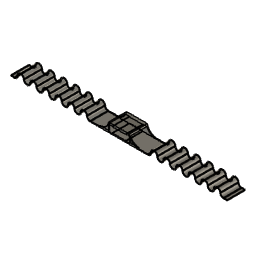
ACUTE_Prototype 3 v1 (Autodesk Fusion 360 design; units mm, degrees)
Autodesk Fusion 360 part; units mm, degrees
note: some values were not read from the file. Set by a fixed rule: which sketch regions a step uses.
sketch "Sketch1" plane through (0, 0, 0) normal (0, 0, 1) x (1, 0, 0)
  line L0 (0, 0) -> (240, 0)
  line L1 (240, 0) -> (240, 20)
  line L2 (240, 20) -> (0, 20)
  line L3 (0, 20) -> (0, 0)
  line L4 (120, 0) -> (120, 20) construction
  line L5 (130, 20) -> (110, 20)
  line L6 (110, 20) -> (110, 0)
  line L7 (110, 0) -> (130, 0)
  line L8 (130, 0) -> (130, 20)
  line L9 (130, 20) -> (110, 0) construction
  line L10 (110, 20) -> (130, 0) construction
  line L11 (127.5, 19) -> (112.5, 19)
  line L12 (112.5, 19) -> (112.5, 1)
  line L13 (112.5, 1) -> (127.5, 1)
  line L14 (127.5, 1) -> (127.5, 19)
  line L15 (127.5, 19) -> (112.5, 1) construction
  line L16 (112.5, 19) -> (127.5, 1) construction
  point P0 (120, 10)
  point P1 (120, 10)
  dimension "d1" = 240
  dimension "d2" = 20
  dimension "d3" = 20
  dimension "d4" = 15
  dimension "d5" = 18
  constraint horizontal L0
  constraint vertical L1
  constraint horizontal L2
  constraint vertical L3
  constraint coincident L0.start L3.end
  constraint midpoint L0 L4.start
  constraint midpoint L2 L4.end
  constraint horizontal L5
  constraint perpendicular L5 L6
  constraint parallel L5 L7
  constraint parallel L6 L8
  constraint coincident L9 P1
  constraint coincident L10 P1
  constraint midpoint L4 P1
  constraint horizontal L11
  constraint perpendicular L11 L12
  constraint parallel L11 L13
  constraint parallel L12 L14
  constraint coincident L15 P1
  constraint coincident L16 P1
  constraint coincident P1 P0
  measures "d1" distance of L0.start L0.end
  measures "d2" distance of L0.start L2.end
  measures "d3" distance of L6.end L7.end
  measures "d4" distance of L12.end L13.end
  measures "d5" distance of L11.end L12.end
extrude "Extrude1" add sketch "Sketch1" along normal blind 10 contours L0 L2 L3 L6 | L0 L2 L5 L6 L7 L8 | L0 L1 L2 L8 | L11 L12 L13 L14
sketch "Sketch2" plane through (0, 0, 0) normal (0, -1, 0) x (1, 0, 0)
  line L0 (0, 0) -> (240, 0)
  line L1 (240, 0) -> (240, 10)
  line L2 (240, 10) -> (0, 10)
  line L3 (0, 10) -> (0, 0)
  line L4 (0, 4) -> (100, 4) construction
  arc A0 (4, 1) -> (7, 4) centre (4, 4) ccw
  arc A1 (4, 0) -> (8, 4) centre (4, 4) ccw
  arc A2 (15, 4) -> (7, 4) centre (11, 4) ccw
  arc A3 (14, 4) -> (8, 4) centre (11, 4) ccw
  arc A4 (14, 4) -> (22, 4) centre (18, 4) ccw
  arc A5 (15, 4) -> (21, 4) centre (18, 4) ccw
  arc A6 (29, 4) -> (21, 4) centre (25, 4) ccw
  arc A7 (28, 4) -> (22, 4) centre (25, 4) ccw
  arc A8 (28, 4) -> (36, 4) centre (32, 4) ccw
  arc A9 (29, 4) -> (35, 4) centre (32, 4) ccw
  arc A10 (43, 4) -> (35, 4) centre (39, 4) ccw
  arc A11 (42, 4) -> (36, 4) centre (39, 4) ccw
  arc A12 (42, 4) -> (50, 4) centre (46, 4) ccw
  arc A13 (43, 4) -> (49, 4) centre (46, 4) ccw
  arc A14 (57, 4) -> (49, 4) centre (53, 4) ccw
  arc A15 (56, 4) -> (50, 4) centre (53, 4) ccw
  arc A16 (56, 4) -> (64, 4) centre (60, 4) ccw
  arc A17 (57, 4) -> (63, 4) centre (60, 4) ccw
  arc A18 (71, 4) -> (63, 4) centre (67, 4) ccw
  arc A19 (70, 4) -> (64, 4) centre (67, 4) ccw
  arc A20 (70, 4) -> (78, 4) centre (74, 4) ccw
  arc A21 (71, 4) -> (77, 4) centre (74, 4) ccw
  arc A22 (85, 4) -> (77, 4) centre (81, 4) ccw
  arc A23 (84, 4) -> (78, 4) centre (81, 4) ccw
  line L5 (0, 0) -> (0, 1) construction
  line L6 (0, 1) -> (98.101, 1) construction
  line L7 (98.101, 1) -> (88, 1)
  arc A24 (85, 4) -> (88, 1) centre (88, 4) ccw
  arc A25 (84, 4) -> (88, 0) centre (88, 4) ccw
  line L8 (4, 1) -> (0, 1)
  line L9 (4, 0) -> (0, 0)
  line L10 (98.101, 1) -> (98.101, 0)
  line L11 (120, 10) -> (120, 0) construction
  line L12 (131.5, 10) -> (108.5, 10)
  line L13 (108.5, 10) -> (108.5, 0)
  line L14 (108.5, 0) -> (131.5, 0)
  line L15 (131.5, 0) -> (131.5, 10)
  line L16 (131.5, 10) -> (108.5, 0) construction
  line L17 (108.5, 10) -> (131.5, 0) construction
  arc A26 (98.101, 1) -> (108.5, 10) centre (98.101, 11.5078) ccw
  point P0 (120, 5)
  dimension "d53" = 4
  dimension "d55" = 8
  dimension "d56" = 6
  dimension "d57" = 8
  dimension "d58" = 6
  dimension "d65" = 1
  dimension "d66" = 8
  dimension "d67" = 6
  dimension "d73" = 23
  constraint coincident L3 L4.start
  constraint concentric A0 A1
  constraint concentric A2 A3
  constraint tangent A0 A2
  constraint tangent A3 A4
  constraint tangent L3 A1
  constraint coincident L4 A0.end
  constraint coincident L4 A1.end
  constraint coincident L4 A3.start
  constraint coincident L4 A5.end
  constraint coincident L4 A2.start
  constraint coincident L4 A4.end
  constraint coincident L4 A7.start
  constraint coincident L4 A6.start
  constraint coincident L4 A9.end
  constraint coincident L4 A8.end
  constraint coincident L4 A11.start
  constraint coincident L4 A10.start
  constraint coincident L4 A13.end
  constraint coincident L4 A12.end
  constraint coincident L4 A15.start
  constraint coincident L4 A14.start
  constraint coincident L4 A17.end
  constraint coincident L4 A16.end
  constraint coincident L4 A19.start
  constraint coincident L4 A18.start
  constraint coincident L4 A21.end
  constraint coincident L4 A20.end
  constraint coincident L4 A23.start
  constraint coincident L4 A22.start
  constraint coincident L0.start L3.end
  constraint perpendicular L5 L6
  constraint concentric A24 A25
  constraint coincident L6 L7.end
  constraint tangent L7 A24
  constraint coincident L0 A25.end
  constraint coincident L6 A0.start
  constraint coincident L0 A1.start
  constraint tangent A0 L8
  constraint tangent A1 L9
  constraint perpendicular L5 L9
  constraint coincident L0 L10.end
  constraint perpendicular L0 L10
  constraint midpoint L2 L11.start
  constraint midpoint L0 L11.end
  constraint horizontal L12
  constraint perpendicular L12 L13
  constraint parallel L12 L14
  constraint parallel L13 L15
  constraint coincident L16 P0
  constraint coincident L17 P0
  constraint midpoint L11 P0
  constraint tangent L7 A26
  measures "d53" distance of L0 L4
  measures "d55" diameter of A1
  measures "d56" diameter of A0
  measures "d57" diameter of A2
  measures "d58" diameter of A3
  measures "d65" distance of L0.start L5.end
  measures "d66" diameter of A25
  measures "d67" diameter of A24
  measures "d73" distance of L13.end L14.end
extrude "Extrude2" cut sketch "Sketch2" against normal blind 30 contours L0 A1 A3 A4 | L2 L3 A0 A2 A5 A6 A9 A10 A13 A14 A17 A18 A21 A22 L7 A24 L8 A26 | L0 A4 A7 A8 | L0 A8 A11 A12 | L0 A12 A15 A16 | L0 A16 A19 A20 | L0 A20 A23 A25
ref_plane "WorkPlane1" through (120, 0, 0) normal (1, 0, 0) x (0, 1, 0)
mirror "Mirror1" about plane through (120, 0, 0) normal (1, 0, 0) of "Extrude2"
sketch "Sketch3" plane through (0, 0, 0) normal (0, -1, 0) x (1, 0, 0)
  arc A0 (152, 0) -> (156, 4) centre (152, 4) ccw
  arc A1 (162, 4) -> (156, 4) centre (159, 4) ccw
  arc A2 (162, 4) -> (170, 4) centre (166, 4) ccw
  arc A3 (176, 4) -> (170, 4) centre (173, 4) ccw
  arc A4 (176, 4) -> (184, 4) centre (180, 4) ccw
  arc A5 (190, 4) -> (184, 4) centre (187, 4) ccw
  arc A6 (190, 4) -> (198, 4) centre (194, 4) ccw
  arc A7 (204, 4) -> (198, 4) centre (201, 4) ccw
  arc A8 (204, 4) -> (212, 4) centre (208, 4) ccw
  arc A9 (218, 4) -> (212, 4) centre (215, 4) ccw
  arc A10 (218, 4) -> (226, 4) centre (222, 4) ccw
  arc A11 (232, 4) -> (226, 4) centre (229, 4) ccw
  arc A12 (232, 4) -> (236, 0) centre (236, 4) ccw
  line L0 (236, 0) -> (240, 0)
  line L1 (240, 0) -> (240, 1)
  line L2 (240, 1) -> (236, 1)
  arc A13 (233, 4) -> (236, 1) centre (236, 4) ccw
  arc A14 (233, 4) -> (225, 4) centre (229, 4) ccw
  arc A15 (219, 4) -> (225, 4) centre (222, 4) ccw
  arc A16 (219, 4) -> (211, 4) centre (215, 4) ccw
  arc A17 (205, 4) -> (211, 4) centre (208, 4) ccw
  arc A18 (205, 4) -> (197, 4) centre (201, 4) ccw
  arc A19 (191, 4) -> (197, 4) centre (194, 4) ccw
  arc A20 (191, 4) -> (183, 4) centre (187, 4) ccw
  arc A21 (177, 4) -> (183, 4) centre (180, 4) ccw
  arc A22 (177, 4) -> (169, 4) centre (173, 4) ccw
  arc A23 (163, 4) -> (169, 4) centre (166, 4) ccw
  arc A24 (163, 4) -> (155, 4) centre (159, 4) ccw
  arc A25 (152, 1) -> (155, 4) centre (152, 4) ccw
  line L3 (152, 1) -> (141.899, 1)
  line L4 (131.5, 10) -> (108.5, 10)
  line L5 (98.101, 1) -> (88, 1)
  arc A26 (85, 4) -> (88, 1) centre (88, 4) ccw
  arc A27 (85, 4) -> (77, 4) centre (81, 4) ccw
  arc A28 (71, 4) -> (77, 4) centre (74, 4) ccw
  arc A29 (71, 4) -> (63, 4) centre (67, 4) ccw
  arc A30 (57, 4) -> (63, 4) centre (60, 4) ccw
  arc A31 (57, 4) -> (49, 4) centre (53, 4) ccw
  arc A32 (43, 4) -> (49, 4) centre (46, 4) ccw
  arc A33 (43, 4) -> (35, 4) centre (39, 4) ccw
  arc A34 (29, 4) -> (35, 4) centre (32, 4) ccw
  arc A35 (29, 4) -> (21, 4) centre (25, 4) ccw
  arc A36 (15, 4) -> (21, 4) centre (18, 4) ccw
  arc A37 (15, 4) -> (7, 4) centre (11, 4) ccw
  arc A38 (4, 1) -> (7, 4) centre (4, 4) ccw
  line L6 (4, 1) -> (0, 1)
  line L7 (0, 1) -> (0, 0)
  line L8 (0, 0) -> (4, 0)
  arc A39 (4, 0) -> (8, 4) centre (4, 4) ccw
  arc A40 (14, 4) -> (8, 4) centre (11, 4) ccw
  arc A41 (14, 4) -> (22, 4) centre (18, 4) ccw
  arc A42 (28, 4) -> (22, 4) centre (25, 4) ccw
  arc A43 (28, 4) -> (36, 4) centre (32, 4) ccw
  arc A44 (42, 4) -> (36, 4) centre (39, 4) ccw
  arc A45 (42, 4) -> (50, 4) centre (46, 4) ccw
  arc A46 (56, 4) -> (50, 4) centre (53, 4) ccw
  arc A47 (56, 4) -> (64, 4) centre (60, 4) ccw
  arc A48 (70, 4) -> (64, 4) centre (67, 4) ccw
  arc A49 (70, 4) -> (78, 4) centre (74, 4) ccw
  arc A50 (84, 4) -> (78, 4) centre (81, 4) ccw
  arc A51 (84, 4) -> (88, 0) centre (88, 4) ccw
  line L9 (88, 0) -> (152, 0)
  arc A52 (131.5, 10) -> (141.899, 1) centre (141.899, 11.5078) ccw
  arc A53 (98.101, 1) -> (108.5, 10) centre (98.101, 11.5078) ccw
sketch "Sketch4" plane through (0, 0, 0) normal (0, -1, 0) x (1, 0, 0)
  line L0 (108.5, 10) -> (131.5, 10) construction
  line L1 (131.5, 10) -> (131.5, 0) construction
  line L2 (131.5, 0) -> (108.5, 0) construction
  line L3 (108.5, 0) -> (108.5, 10) construction
  line L4 (88, 0) -> (152, 0)
  line L5 (108.5, 0) -> (131.5, 0) construction
  line L6 (131.5, 0) -> (131.5, 1) construction
  line L7 (131.5, 1) -> (108.5, 1) construction
  line L8 (108.5, 1) -> (108.5, 0) construction
  line L9 (108.5, 1) -> (131.5, 1) construction
  line L10 (131.5, 1) -> (131.5, 1.5) construction
  line L11 (131.5, 1.5) -> (108.5, 1.5)
  line L12 (108.5, 1.5) -> (108.5, 1) construction
  line L13 (131.5, 1.5) -> (108.5, 1.5)
  line L14 (108.5, 1.5) -> (108.5, 7.5)
  line L15 (108.5, 7.5) -> (131.5, 7.5)
  line L16 (131.5, 7.5) -> (131.5, 1.5)
  line L17 (127.5006, 1) -> (112.5006, 1)
  line L18 (112.5006, 1) -> (112.5006, 1.5)
  line L19 (127.5006, 1.5) -> (127.5006, 1)
  line L20 (127.5006, 1) -> (120, 1.5) construction
  line L21 (112.5006, 1) -> (120, 1.5) construction
  line L22 (112.5, 7.5) -> (112.5, 8)
  line L23 (112.5, 8) -> (127.5, 8)
  line L24 (127.5, 8) -> (127.5, 7.5)
  line L25 (120, 7.5) -> (112.5, 8) construction
  line L26 (120, 7.5) -> (127.5, 8) construction
  line L27 (127.5, 7.5) -> (127.5, 1.5) construction
  line L28 (127.5, 8) -> (131.5, 8)
  line L29 (131.5, 8) -> (131.5, 7.5)
  line L30 (112.5, 8) -> (108.5, 8)
  line L31 (108.5, 8) -> (108.5, 7.5)
  line L32 (108.5, 1.5) -> (108.5, 1)
  line L33 (112.5006, 1) -> (108.5, 1)
  line L34 (131.5, 1.5) -> (131.5, 1)
  line L35 (131.5, 1) -> (127.5006, 1)
  point P0 (108.5, 10)
  dimension "d74" = 1
  dimension "d75" = 0.5
  dimension "d76" = 6
  dimension "d78" = 15
  dimension "d80" = 0.5
  dimension "d81" = 15
  constraint horizontal L0
  constraint vertical L1
  constraint horizontal L2
  constraint vertical L3
  constraint coincident L1.end L4
  constraint coincident P0 L0.start
  constraint horizontal L5
  constraint vertical L6
  constraint horizontal L7
  constraint vertical L8
  constraint horizontal L9
  constraint vertical L10
  constraint horizontal L11
  constraint vertical L12
  constraint horizontal L13
  constraint vertical L14
  constraint horizontal L15
  constraint vertical L16
  constraint horizontal L17
  constraint perpendicular L17 L18
  constraint parallel L18 L19
  constraint coincident L7 L17.start
  constraint midpoint L11 L20.end
  constraint coincident L11 L19.start
  constraint coincident L11 L18.end
  constraint parallel L22 L24
  constraint midpoint L15 L25.start
  constraint coincident L15 L22.start
  constraint coincident L15 L24.end
  constraint coincident L11 L27.end
  constraint perpendicular L11 L27
  constraint coincident L1 L28.end
  constraint perpendicular L1 L28
  constraint perpendicular L15 L29
  constraint coincident L3 L30.end
  constraint perpendicular L3 L30
  constraint perpendicular L15 L31
  constraint perpendicular L7 L34
  constraint perpendicular L19 L35
  measures "d74" distance of L2.end L7.end
  measures "d75" distance of L7.end L11.end
  measures "d76" distance of L10.end L15.end
  measures "d78" distance of L22.end L23.end
  measures "d80" distance of L22.end L22.start
  measures "d81" distance of L18 L19
extrude "Extrude3" cut sketch "Sketch4" against normal blind 19 contours L11 L13 L19 L34 L35 | L11 L13 L14 L15 L16 | L15 L24 L28 L29 | L11 L13 L18 L32 L33 | L15 L22 L30 L31
sketch "Sketch5" plane through (108.5, 0, 0) normal (1, 0, 0) x (0, 1, 0)
  line L0 (0, 8) -> (0, 1)
  line L1 (0, 1) -> (19, 1)
  line L2 (19, 1) -> (19, 8)
  line L3 (19, 8) -> (0, 8)
  line L4 (19, 8) -> (1, 8)
  line L5 (1, 8) -> (1, 1)
  line L6 (1, 1) -> (19, 1)
  line L7 (19, 1) -> (19, 8)
  dimension "d84" = 18
  constraint horizontal L4
  constraint vertical L5
  constraint horizontal L6
  constraint vertical L7
  constraint coincident L2.end L3.start
  measures "d84" distance of L2.end L4.end
extrude "Extrude4" cut sketch "Sketch5" against normal blind 12 contours L1 L2 L3 L4 L5 L6 L7
sketch "Sketch6" plane through (131.5, 0, 0) normal (-1, 0, 0) x (0, -1, 0)
  line L0 (0, 1) -> (0, 8)
  line L1 (0, 8) -> (-19, 8)
  line L2 (-19, 8) -> (-19, 1)
  line L3 (-19, 1) -> (0, 1)
  line L4 (-19, 1) -> (-1, 1)
  line L5 (-1, 1) -> (-1, 8)
  line L6 (-1, 8) -> (-19, 8)
  line L7 (-19, 8) -> (-19, 1)
  dimension "d87" = 18
  constraint horizontal L4
  constraint vertical L5
  constraint horizontal L6
  constraint vertical L7
  constraint coincident L2.end L3.start
  measures "d87" distance of L2.end L4.end
extrude "Extrude5" cut sketch "Sketch6" against normal blind 11 contours L1 L2 L3 L4 L5 L6 L7
sketch "Sketch7" plane through (0, 0, 0) normal (0, -1, 0) x (1, 0, 0)
  line L0 (112.5, 7.5) -> (127.5, 7.5)
  line L1 (127.5, 7.5) -> (127.5, 8)
  line L2 (127.5, 8) -> (131.5, 8)
  line L3 (131.5, 8) -> (131.5, 1)
  line L4 (131.5, 1) -> (127.5006, 1)
  line L5 (127.5006, 1) -> (127.5006, 1.5)
  line L6 (127.5006, 1.5) -> (112.5006, 1.5)
  line L7 (112.5006, 1.5) -> (112.5006, 1)
  line L8 (112.5006, 1) -> (108.5, 1)
  line L9 (108.5, 1) -> (108.5, 8)
  line L10 (108.5, 8) -> (112.5, 8)
  line L11 (112.5, 8) -> (112.5, 7.5)
  arc A0 (152, 0) -> (156, 4) centre (152, 4) ccw
  arc A1 (162, 4) -> (156, 4) centre (159, 4) ccw
  arc A2 (162, 4) -> (170, 4) centre (166, 4) ccw
  arc A3 (176, 4) -> (170, 4) centre (173, 4) ccw
  arc A4 (176, 4) -> (184, 4) centre (180, 4) ccw
  arc A5 (190, 4) -> (184, 4) centre (187, 4) ccw
  arc A6 (190, 4) -> (198, 4) centre (194, 4) ccw
  arc A7 (204, 4) -> (198, 4) centre (201, 4) ccw
  arc A8 (204, 4) -> (212, 4) centre (208, 4) ccw
  arc A9 (218, 4) -> (212, 4) centre (215, 4) ccw
  arc A10 (218, 4) -> (226, 4) centre (222, 4) ccw
  arc A11 (232, 4) -> (226, 4) centre (229, 4) ccw
  arc A12 (232, 4) -> (236, 0) centre (236, 4) ccw
  line L12 (236, 0) -> (240, 0)
  line L13 (240, 0) -> (240, 1)
  line L14 (240, 1) -> (236, 1)
  arc A13 (233, 4) -> (236, 1) centre (236, 4) ccw
  arc A14 (233, 4) -> (225, 4) centre (229, 4) ccw
  arc A15 (219, 4) -> (225, 4) centre (222, 4) ccw
  arc A16 (219, 4) -> (211, 4) centre (215, 4) ccw
  arc A17 (205, 4) -> (211, 4) centre (208, 4) ccw
  arc A18 (205, 4) -> (197, 4) centre (201, 4) ccw
  arc A19 (191, 4) -> (197, 4) centre (194, 4) ccw
  arc A20 (191, 4) -> (183, 4) centre (187, 4) ccw
  arc A21 (177, 4) -> (183, 4) centre (180, 4) ccw
  arc A22 (177, 4) -> (169, 4) centre (173, 4) ccw
  arc A23 (163, 4) -> (169, 4) centre (166, 4) ccw
  arc A24 (163, 4) -> (155, 4) centre (159, 4) ccw
  arc A25 (152, 1) -> (155, 4) centre (152, 4) ccw
  line L15 (152, 1) -> (141.899, 1)
  arc A26 (131.5, 10) -> (141.899, 1) centre (141.899, 11.5078) ccw
  line L16 (131.5, 10) -> (108.5, 10)
  arc A27 (98.101, 1) -> (108.5, 10) centre (98.101, 11.5078) ccw
  line L17 (98.101, 1) -> (88, 1)
  arc A28 (85, 4) -> (88, 1) centre (88, 4) ccw
  arc A29 (85, 4) -> (77, 4) centre (81, 4) ccw
  arc A30 (71, 4) -> (77, 4) centre (74, 4) ccw
  arc A31 (71, 4) -> (63, 4) centre (67, 4) ccw
  arc A32 (57, 4) -> (63, 4) centre (60, 4) ccw
  arc A33 (57, 4) -> (49, 4) centre (53, 4) ccw
  arc A34 (43, 4) -> (49, 4) centre (46, 4) ccw
  arc A35 (43, 4) -> (35, 4) centre (39, 4) ccw
  arc A36 (29, 4) -> (35, 4) centre (32, 4) ccw
  arc A37 (29, 4) -> (21, 4) centre (25, 4) ccw
  arc A38 (15, 4) -> (21, 4) centre (18, 4) ccw
  arc A39 (15, 4) -> (7, 4) centre (11, 4) ccw
  arc A40 (4, 1) -> (7, 4) centre (4, 4) ccw
  line L18 (4, 1) -> (0, 1)
  line L19 (0, 1) -> (0, 0)
  line L20 (0, 0) -> (4, 0)
  arc A41 (4, 0) -> (8, 4) centre (4, 4) ccw
  arc A42 (14, 4) -> (8, 4) centre (11, 4) ccw
  arc A43 (14, 4) -> (22, 4) centre (18, 4) ccw
  arc A44 (28, 4) -> (22, 4) centre (25, 4) ccw
  arc A45 (28, 4) -> (36, 4) centre (32, 4) ccw
  arc A46 (42, 4) -> (36, 4) centre (39, 4) ccw
  arc A47 (42, 4) -> (50, 4) centre (46, 4) ccw
  arc A48 (56, 4) -> (50, 4) centre (53, 4) ccw
  arc A49 (56, 4) -> (64, 4) centre (60, 4) ccw
  arc A50 (70, 4) -> (64, 4) centre (67, 4) ccw
  arc A51 (70, 4) -> (78, 4) centre (74, 4) ccw
  arc A52 (84, 4) -> (78, 4) centre (81, 4) ccw
  arc A53 (84, 4) -> (88, 0) centre (88, 4) ccw
  line L21 (88, 0) -> (152, 0)
equation "d57 = d55"
equation "d58 = d56"
equation "d66 = d55"
equation "d67 = d56"
